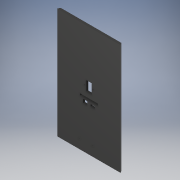
# Autodesk Inventor part: BA03
Saved by Autodesk Inventor 2017 (Build 210142000, 142)
## iProperties
Created: 2018-10-18
Part Number: BA03
Material: ABS Plastic
Document SubType Name: Modeling
Designer: Dell
Density: 1.06 g/cm^3
Appearance: Smooth - Black
Author: Dell
Autodesk Inventor part; units mm, degrees
ref_plane "YZ Plane" through (0, 0, 0) normal (1, 0, 0) x (0, 1, 0)
ref_plane "XZ Plane" through (0, 0, 0) normal (0, 1, 0) x (-1, 0, 0)
ref_plane "XY Plane" through (0, 0, 0) normal (0, 0, 1) x (1, 0, 0)
sketch "Sketch1" plane through (0, 0, 0) normal (0, 0, 1) x (1, 0, 0)
  line L0 (0, 0) -> (292.1, 0)
  line L1 (292.1, 0) -> (292.1, -533.4)
  line L2 (292.1, -533.4) -> (0, -533.4)
  line L3 (0, -533.4) -> (0, 0)
  dimension "d0" = 292.1
  dimension "d1" = 533.4
  constraints: 8 end point, 2 parallel, 1 horizontal, 1 perpendicular
  measures "d0" distance of L1.end L2.end
  measures "d1" distance of L0.end L1.end
extrude "Extrusion1" add sketch "Sketch1" along normal blind 10
sketch "Sketch2" plane through (0, 0, 0) normal (0, 1, 0) x (1, 0, 0)
  line L0 (292.1, -10) -> (0, -10) projected
  line L1 (0, -10) -> (-5.7735, -10)
  line L2 (-5.7735, -10) -> (0, 0)
  line L3 (0, 0) -> (0, -10) projected
  line L4 (0, 0) -> (0, -10) projected
  line L5 (0, -10) -> (0, 0)
  line L6 (292.1, -10) -> (297.8735, -10)
  line L7 (292.1, 0) -> (292.1, -10) projected
  line L8 (297.8735, -10) -> (292.1, 0)
  line L9 (292.1, 0) -> (292.1, -10)
  dimension "d4" = 30
  dimension "d5" = 60
  constraints: 12 end point, 2 collinear, 2 horizontal
  measures "d4" angle of L3 L2
  measures "d5" angle of L6 L8
extrude "Extrusion2" add sketch "Sketch2" against normal blind 533.4
sketch "Sketch4" plane through (0, 0, 10) normal (0, 0, 1) x (1, 0, 0)
  line L0 (132.05, -228.6) -> (160.05, -228.6)
  line L1 (160.05, -228.6) -> (160.05, -278.6)
  line L2 (160.05, -278.6) -> (132.05, -278.6)
  line L3 (132.05, -278.6) -> (132.05, -228.6)
  line L4 (-5.7735, 0) -> (-5.7735, -533.4) projected
  line L5 (-5.7735, 0) -> (297.8735, 0) projected
  line L6 (297.8735, -533.4) -> (-5.7735, -533.4) projected
  circle A0 centre (126.05, -253.6) radius 3
  circle A1 centre (166.05, -253.6) radius 3
  point P0 (0, 0)
  point P1 (146.05, -228.6)
  point P2 (146.05, 0)
  point P3 (160.05, -253.6)
  point P4 (132.05, -253.6)
  dimension "d16" = 28
  dimension "d17" = 50
  dimension "d19" = 6
  dimension "d20" = 6
  dimension "d21" = 6
  dimension "d22" = 6
  dimension "d41" = 228.6
  constraints: 8 end point, 4 midpoint, 2 centre point, 2 horizontal alignment, 2 parallel, 1 horizontal, 1 perpendicular, 1 vertical alignment
  measures "d16" distance of L1.end L2.end
  measures "d17" distance of L0.end L1.end
  measures "d19" diameter of A0
  measures "d20" diameter of A1
  measures "d21" distance from line of L3 A0.centre
  measures "d22" distance from line of A1.centre L1
  measures "d41" distance between parallel lines of L5 L0
extrude "Extrusion4" cut sketch "Sketch4" against normal through all
sketch "Sketch5" plane through (0, 0, 10) normal (0, 0, 1) x (1, 0, 0)
  line L0 (189.55, -309.6) -> (102.55, -309.6)
  line L1 (102.55, -309.6) -> (102.55, -298.6)
  line L2 (102.55, -298.6) -> (189.55, -298.6)
  line L3 (189.55, -298.6) -> (189.55, -309.6)
  line L4 (160.05, -278.6) -> (132.05, -278.6) projected
  line L5 (175.55, -330.6) -> (153.55, -330.6)
  line L6 (153.55, -330.6) -> (153.55, -318.6)
  line L7 (153.55, -318.6) -> (175.55, -318.6)
  line L8 (175.55, -318.6) -> (175.55, -330.6)
  line L9 (138.55, -334.6) -> (116.55, -334.6)
  line L10 (116.55, -334.6) -> (116.55, -314.6)
  line L11 (116.55, -314.6) -> (138.55, -314.6)
  line L12 (138.55, -314.6) -> (138.55, -334.6)
  line L13 (153.55, -324.6) -> (138.55, -324.6) construction
  point P0 (0, 0)
  point P1 (146.05, -298.6)
  point P2 (146.05, -278.6)
  point P3 (146.05, -324.6)
  dimension "d26" = 87
  dimension "d27" = 11
  dimension "d28" = 20
  dimension "d29" = 22
  dimension "d30" = 12
  dimension "d32" = 22
  dimension "d33" = 20
  dimension "d37" = 15
  dimension "d38" = 15
  constraints: 26 end point, 6 parallel, 5 midpoint, 4 horizontal, 3 perpendicular, 2 vertical alignment, 1 horizontal alignment
  measures "d26" distance of L1.end L2.end
  measures "d27" distance of L0.end L1.end
  measures "d28" distance between parallel lines of L4 L2
  measures "d29" distance of L6.end L7.end
  measures "d30" distance of L5.end L6.end
  measures "d32" distance of L10.end L11.end
  measures "d33" distance of L9.end L10.end
  measures "d37" distance from line of L0 L13.start
  measures "d38" distance between parallel lines of L12 L6
extrude "Extrusion5" cut sketch "Sketch5" against normal through all
sketch "Sketch6" plane through (0, 0, 10) normal (0, 0, 1) x (1, 0, 0)
  circle A0 centre (164.5, -488.95) radius 2.3812
  circle A1 centre (101, -488.95) radius 2.3813
  line L0 (0, -533.4) -> (0, 0) projected
  line L1 (292.1, -533.4) -> (0, -533.4) projected
  dimension "d42" = 101
  dimension "d43" = 44.45
  dimension "d44" = 4.7625
  dimension "d45" = 4.7625
  dimension "d46" = 63.5
  constraints: 2 centre point, 1 horizontal alignment
  measures "d42" distance from line of L0 A1.centre
  measures "d43" distance from line of L1 A1.centre
  measures "d44" diameter of A1
  measures "d45" diameter of A0
  measures "d46" distance of A0.centre A1.centre
extrude "Extrusion6" cut sketch "Sketch6" against normal through all
body "Solid1"
